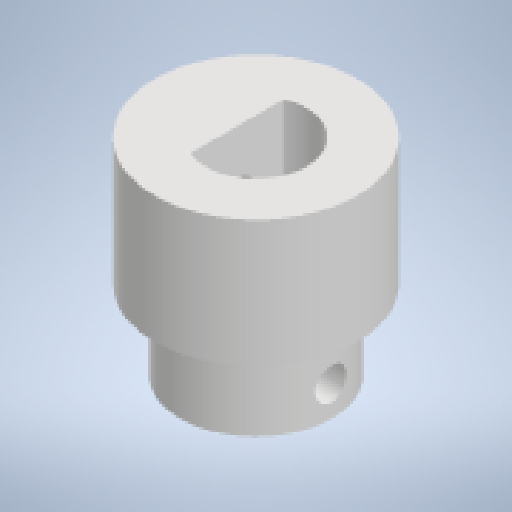
# Autodesk Inventor part: Acople2
Saved by Autodesk Inventor 2023 (Build 270158000, 158)
## iProperties
Created: 2022-12-24
Part Number: Acople2
Material: Genérico
Document SubType Name: Modeling
Designer: sergi
Density: 1 g/cm^3
Appearance: Valor por defecto
Author: sergi
Autodesk Inventor part; units mm, degrees
ref_plane "YZ Plane" through (0, 0, 0) normal (1, 0, 0) x (0, 1, 0)
ref_plane "XZ Plane" through (0, 0, 0) normal (0, 1, 0) x (-1, 0, 0)
ref_plane "XY Plane" through (0, 0, 0) normal (0, 0, 1) x (1, 0, 0)
sketch "Boceto1" plane through (0, 0, 0) normal (0, 1, 0) x (-1, 0, 0)
  circle A0 centre (0, 0) radius 8
  circle A1 centre (0, 0) radius 4
  dimension "d0" = 16
  dimension "d1" = 8
  constraints: 2 centre point, 2 coincident
  measures "d0" diameter of A0
  measures "d1" diameter of A1
extrude "Extrusión1" add sketch "Boceto1" along normal blind 10 contours A0 | A1
sketch "Boceto2" plane through (0, 0, 0) normal (1, 0, 0) x (0, 1, 0)
  line L0 (0, 0) -> (5, 0)
  circle A0 centre (5, 0) radius 1.5
  dimension "d4" = 5
  dimension "d5" = 3
  constraints: 2 end point, 1 centre point, 1 coincident, 1 horizontal
  measures "d4" distance of L0.start L0.end
  measures "d5" diameter of A0
hole "Agujero1" at (0, 5, 0) direction (-1, 0, 0) diameter 3 end through all
sketch "Boceto4" plane through (0, 10, 0) normal (0, 1, 0) x (1, 0, 0)
  circle A0 centre (0, 0) radius 4
  line L0 (0, 4) -> (0, -4)
  line L1 (-1.5, 4) -> (-1.5, -4)
  point P0 (-1.5, 3.7081)
  point P1 (-1.5, -3.7081)
  dimension "d21" = 8
  dimension "d45" = 1.5
  constraints: 4 end point, 2 point on circle, 1 centre point, 1 coincident, 1 parallel, 1 vertical
  measures "d21" diameter of A0
  measures "d45" distance between parallel lines of L0 L1
extrude "Extrusión2" cut sketch "Boceto4" against normal blind 8 contours A0 L0 | L0 A0 L1
sketch "Boceto5" plane through (0, 0, 0) normal (0, -1, 0) x (1, 0, 0)
  circle A0 centre (0, 0) radius 6
  dimension "d24" = 12
  constraints: 1 centre point, 1 coincident
  measures "d24" diameter of A0
extrude "Extrusión3" add sketch "Boceto5" along normal blind 6.25
sketch "Boceto8" plane through (0, -6.25, 0) normal (0, -1, 0) x (1, 0, 0)
  circle A0 centre (0, 0) radius 1.75
  line L0 (1, 0) -> (-1, 0) projected
  line L1 (1.75, 0) -> (1, 0)
  line L2 (1, 0) -> (1, 1.5)
  line L3 (1, 1.5) -> (1, -2.7879)
  point P0 (1, -1.4361)
  point P1 (1, 1.4361)
  dimension "d46" = 3.5
  dimension "d47" = 0.75
  constraints: 6 end point, 1 coincident, 1 collinear, 1 perpendicular, 1 point on line, 3 other
  measures "d47" distance of L1.start L0.start
extrude "Extrusión6" cut sketch "Boceto8" against normal blind 8.25 contours L2 L3 A0
sketch "Boceto9" plane through (0, -6.25, 0) normal (0, -1, 0) x (1, 0, 0)
  circle A0 centre (0, 0) radius 1.5
  constraints: 1 centre point, 1 coincident
extrude "Extrusión7" cut sketch "Boceto9" against normal blind 1.4
ref_plane "Plano de trabajo1" through (-8, 10, 3.7081) normal (1, 0, 0) x (0, 0, -1)
sketch "Boceto10" plane through (-8, 10, 3.7081) normal (1, 0, 0) x (0, 0, -1)
  spline S0 degree 2 poles (5.2081, -5) (5.2081, -7.5981) (2.9581, -6.299) (0.7081, -5) (2.9581, -3.701) (5.2081, -2.4019) (5.2081, -5) knots 0 0 0 0.333333 0.333333 0.666667 0.666667 1 1 1 weights 1 0.5 1 0.5 1 0.5 1 projected
  circle A0 centre (3.7081, -5) radius 3
  point P0 (3.7081, -10)
  dimension "d53" = 6
  constraints: 1 centre point, 1 other
  measures "d53" diameter of A0
extrude "Extrusión8" cut sketch "Boceto10" along normal blind 2
sketch "Boceto11" plane through (0, 0, 0) normal (1, 0, 0) x (0, 1, 0)
  line L0 (-1.5, 0) -> (-1.5, 2.5882)
  line L1 (-1.5, 0) -> (-1.5, 2.5882)
  line L2 (0, 0) -> (-1.5, 0)
  line L3 (-4.85, -1.118) -> (-4.85, 1.118) projected
  line L4 (-1.5, -4) -> (-1.5, 4)
  line L5 (-6.25, 6) -> (-6.25, -6) projected
  line L6 (-1.5, 0) -> (-6.25, 0)
  circle A0 centre (-3.875, 0) radius 1.25
  dimension "d59" = 2.5
  constraints: 10 end point, 3 vertical, 2 midpoint, 1 centre point, 1 horizontal, 4 other
  measures "d59" diameter of A0
extrude "Extrusión9" cut sketch "Boceto11" along normal through all
